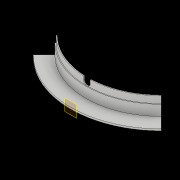
# Autodesk Inventor part: Layer2_Bottom_Quarter
Saved by Autodesk Inventor 2017 (Build 210142000, 142)
## iProperties
Created: 2017-01-16
Part Number: Layer2_Bottom_Quarter
Material: Generic
Document SubType Name: Modeling
Designer: David Kopala
Density: 1 g/cm^3
Appearance: Default
Author: David Kopala
Autodesk Inventor part; units mm, degrees
ref_plane "YZ Plane" through (0, 0, 0) normal (1, 0, 0) x (0, 1, 0)
ref_plane "XZ Plane" through (0, 0, 0) normal (0, 1, 0) x (-1, 0, 0)
ref_plane "XY Plane" through (0, 0, 0) normal (0, 0, 1) x (1, 0, 0)
sketch "Sketch1" plane through (0, 0, 0) normal (1, 0, 0) x (0, 1, 0)
  line L0 (0, 0) -> (50.8, 0)
  line L1 (0, 138.1125) -> (26.719, 138.1125)
  line L2 (0, 138.1125) -> (0, 169.8625)
  line L3 (0, 169.8625) -> (3.175, 169.8625)
  line L4 (3.175, 169.8625) -> (3.175, 141.2875)
  line L5 (3.175, 141.2875) -> (22.9489, 141.2875)
  line L6 (60.325, 141.2875) -> (60.325, 179.3875)
  line L7 (60.325, 179.3875) -> (63.5, 179.3875)
  line L8 (63.5, 179.3875) -> (63.5, 138.1125)
  line L9 (35.6489, 138.1125) -> (26.719, 138.1125)
  line L10 (29.2989, 139.7) -> (22.9489, 139.7)
  line L11 (22.9489, 139.7) -> (22.9489, 141.2875)
  line L12 (29.2989, 139.7) -> (35.6489, 139.7)
  line L13 (35.6489, 139.7) -> (35.6489, 138.1125)
  line L14 (29.2989, 166.1379) -> (29.2989, 141.2875)
  line L15 (29.2989, 138.1125) -> (29.2989, 120.1049)
  point P0 (62.1333, 179.3875)
  point P1 (1.5875, 169.8625)
  dimension "d0" = 50.8
  dimension "d1" = 138.1125
  dimension "d2" = 31.75
  dimension "d3" = 3.175
  dimension "d4" = 3.175
  dimension "d5" = 57.15
  dimension "d6" = 38.1
  dimension "d7" = 3.175
  dimension "d13" = 26.1239
  dimension "d14" = 1.5875
  dimension "d15" = 6.35
  dimension "d16" = 6.35
  constraints: 32 end point, 6 perpendicular, 4 horizontal, 4 point on line, 3 vertical, 1 collinear, 1 midpoint, 1 parallel
  measures "d0" distance of L0.start L0.end
  measures "d1" distance between parallel lines of L0 L1
  measures "d2" distance of L1.start L2.end
  measures "d3" distance of L2.end L3.end
  measures "d4" distance from line of L1 L4.end
  measures "d5" distance of L4.end L6.start
  measures "d6" distance of L6.start L6.end
  measures "d7" distance of L6.end L7.end
  measures "d13" distance from line of L14.start L4
  measures "d14" distance from line of L9 L10.start
  measures "d15" distance of L10.start L10.end
  measures "d16" distance of L10.start L12.end
revolve "Revolution1" add sketch "Sketch1" angle 360 about axis through (0, 0, 0) along (0, 1, 0)
ref_plane "Work Plane2" through (0, 1.5875, 169.8625) normal (0, 0, 1) x (1, 0, 0)
sketch "Sketch3" plane through (0, 1.5875, 169.8625) normal (0, 0, 1) x (1, 0, 0)
  arc A0 (-6.3749, 27.6865) -> (6.3749, 27.6865) centre (0, 27.6865) ccw
  line L0 (138.1125, 34.0614) -> (-138.1125, 34.0614) projected
  line L1 (-6.3749, 27.6865) -> (-6.3749, 34.0614)
  line L2 (6.3749, 27.6865) -> (6.3749, 34.0614)
  point P0 (0, -1.5875)
  point P1 (0, 17.4621)
  constraints: 4 end point, 3 tangent, 2 point on circle, 2 point on line, 1 centre point, 1 perpendicular, 1 vertical
extrude "Extrusion2" cut sketch "Sketch3" against normal through all
sketch "Sketch4" plane through (0, 0, 0) normal (0, -1, 0) x (1, 0, 0)
  line L0 (0, 0) -> (-198.1259, 198.1259)
  line L1 (0, 0) -> (280.1923, 0) construction
  line L2 (-198.1259, 198.1259) -> (-198.1259, -227.7187)
  line L3 (-198.1259, -227.7187) -> (214.1573, -227.7187)
  line L4 (0, 0) -> (198.1259, 198.1259)
  line L5 (198.1259, 198.1259) -> (214.1573, -227.7187)
  dimension "d19" = 135
  dimension "d20" = 90
  constraints: 12 end point, 1 equal length, 1 horizontal, 1 perpendicular, 1 vertical
  measures "d19" angle of L1 L0
  measures "d20" angle of L0 L4
extrude "Extrusion3" cut sketch "Sketch4" against normal through all
body "Solid1"
